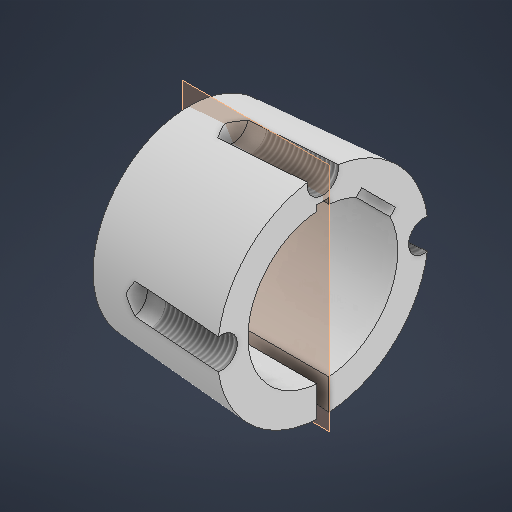
# Autodesk Inventor part: Douille1008
Saved by Autodesk Inventor 2026.2 (Build 302298010, 298A)
## iProperties
Created: 2026-04-10
Part Number: Douille1008
Material: Générique
Document SubType Name: Modeling
Designer: romai
Density: 1 g/cm^3
Appearance: Par défaut
Author: romai
Autodesk Inventor part; units mm, degrees
ref_plane "YZ Plane" through (0, 0, 0) normal (1, 0, 0) x (0, 1, 0)
ref_plane "XZ Plane" through (0, 0, 0) normal (0, 1, 0) x (-1, 0, 0)
sketch "Esquisse1" plane through (0, 0, 0) normal (0, 0, 1) x (1, 0, 0)
  line L0 (-36.1898, 0) -> (37.2521, 0)
  line L1 (0, 12.5) -> (-22.3, 12.5)
  line L2 (-22.3, 12.5) -> (-22.3, 16)
  line L3 (-22.3, 16) -> (0, 17.6)
  line L4 (0, 17.6) -> (0, 12.5)
  point P0 (0, 0)
  dimension "d0" = 25
  dimension "d1" = 35.2
  dimension "d2" = 0
  dimension "d3" = 32
  dimension "d4" = 22.3
  dimension "d5" = 0
  constraints: 10 end point, 2 horizontal, 1 parallel, 1 perpendicular
  measures "d0" diameter of L1 L0
  measures "d1" diameter of L3.end L0
  measures "d2" distance from line of point (0, 0) L0
  measures "d3" diameter of L2.end L0
  measures "d4" distance between parallel lines of L4 L2
  measures "d5" distance from line of point (0, 0) L4
revolve "Révolution1" add sketch "Esquisse1" angle 360 about axis through (-36.1898, 0, 0) along (1, 0, 0)
sketch "Esquisse4" plane through (0, 0, 0) normal (1, 0, 0) x (0, 0, 1)
  line L0 (0, 0) -> (-39.036, -39.036)
  line L1 (0, 0) -> (-55.3193, 0)
  circle A0 centre (0, 0) radius 12.5 projected
  line L2 (-5.5456, -11.2025) -> (-6.4649, -12.1217)
  line L3 (-11.2025, -5.5456) -> (-12.1217, -6.4649)
  line L4 (-12.1217, -6.4649) -> (-6.4649, -12.1217)
  dimension "d17" = 45
  dimension "d20" = 1.3
  dimension "d21" = 1.3
  dimension "d22" = 4
  dimension "d23" = 4
  constraints: 10 end point, 2 parallel, 2 point on circle, 1 horizontal
  measures "d17" angle of L1 L0
  measures "d20" distance of L2.start L2.end
  measures "d21" distance of L3.start L3.end
  measures "d22" distance between parallel lines of L0 L3
  measures "d23" distance between parallel lines of L0 L2
extrude "Extrusion1" cut sketch "Esquisse4" against normal through all contours A0 L2 L4 L0 | L0 L4 L3 A0
sketch "Esquisse5" plane through (0, 0, 0) normal (1, 0, 0) x (0, 0, 1)
  line L0 (-1, 17.6) -> (1, 17.6)
  line L1 (1, 17.6) -> (1, -13.4)
  line L2 (1, -13.4) -> (-1, -13.4)
  line L3 (-1, -13.4) -> (-1, 17.6)
  line L4 (-1, 17.6) -> (1, -13.4) construction
  line L5 (1, 17.6) -> (-1, -13.4) construction
  arc A0 (0, -17.6) -> (0, -17.6) centre (0, 0) ccw projected
  point P0 (0, 2.1)
  dimension "d26" = 2
  dimension "d27" = 31
  dimension "d28" = 0
  constraints: 12 end point, 2 midpoint, 2 parallel, 1 horizontal, 1 perpendicular, 1 tangent
  measures "d26" distance of L1.end L2.end
  measures "d27" distance of L0.end L1.end
  measures "d28" horizontal distance of point (0, 0) point (0, 2.1)
extrude "Extrusion2" cut sketch "Esquisse5" against normal through all contours L0 A0 L3 | L0 L1 A0 | A0 L1 L2 L3 picked at (0, -3.0667)
sketch "Esquisse6" plane through (0, 0, 0) normal (1, 0, 0) x (0, 0, -1)
  line L0 (0, 0) -> (0, 23.579)
  line L1 (0, 0) -> (-21.6871, 0)
  line L2 (0, 0) -> (25.1017, 0)
  circle A0 centre (0, 0) radius 16.865
  point P0 (0, 16.865)
  point P1 (16.865, 0)
  point P2 (-16.865, 0)
  dimension "d39" = 33.73
  constraints: 6 end point, 3 point on circle, 3 point on line, 2 horizontal, 1 centre point, 1 coincident, 1 vertical
  measures "d39" diameter of A0
hole "Perçage2" at (0, 16.865, 0) at (0, 0, -16.865) at (0, 0, 16.865) direction (-1, 0, 0) diameter 5.1881 depth 15 tip angle 118 thread size "M6x0.75" class "6H" standard "ANSI Metric M Profile"
